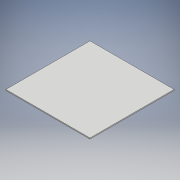
# Autodesk Inventor part: mainboard
Saved by Autodesk Inventor 2017 (Build 210142000, 142)
## iProperties
Created: 2017-06-07
Part Number: mainboard
Material: Generic
Document SubType Name: Modeling
Designer: Roko
Density: 1 g/cm^3
Appearance: Default
Author: Roko
Autodesk Inventor part; units mm, degrees
ref_plane "YZ Plane" through (0, 0, 0) normal (1, 0, 0) x (0, 1, 0)
ref_plane "XZ Plane" through (0, 0, 0) normal (0, 1, 0) x (-1, 0, 0)
ref_plane "XY Plane" through (0, 0, 0) normal (0, 0, 1) x (1, 0, 0)
sketch "Sketch1" plane through (0, 0, 0) normal (0, 0, 1) x (1, 0, 0)
  line L0 (-122, -122) -> (122, -122)
  line L1 (122, -122) -> (122, 122)
  line L2 (122, 122) -> (-122, 122)
  line L3 (-122, 122) -> (-122, -122)
  line L4 (-122, -122) -> (122, 122) construction
  line L5 (122, -122) -> (-122, 122) construction
  point P0 (0, 0)
  dimension "d0" = 244
  dimension "d1" = 244
  constraints: 12 end point, 2 midpoint, 2 parallel, 1 horizontal, 1 perpendicular
  measures "d0" distance of L2.end L1.end
  measures "d1" distance of L1.end L0.end
extrude "Extrusion1" add sketch "Sketch1" along normal blind 3
body "Solid1"
